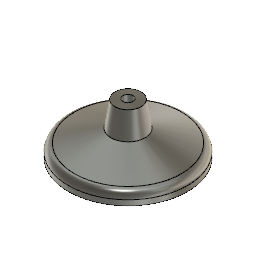
flag support (Autodesk Fusion 360 design; units mm, degrees)
Autodesk Fusion 360 part; units mm, degrees
sketch "Sketch1" plane through (0, 0, 0) normal (0, 1, 0) x (1, 0, 0)
  line L0 (0, -65) -> (0, 55)
  line L1 (-35, 24.9628) -> (-1, 24.9628)
  line L2 (-35, 24.9628) -> (-35, 21.7628)
  arc A0 (-35, 21.7628) -> (-31.4072, 17.5424) centre (-30.7249, 21.7628) ccw
  line L3 (-31.4072, 17.5424) -> (-10, 10)
  line L4 (-10, 10) -> (-7.7084, -4.6955)
  line L5 (0, -5) -> (-3, -5) construction
  line L6 (-7.7084, -4.6955) -> (-3, -5)
  line L7 (-3, -5) -> (-3, 20)
  line L8 (-1, 24.9628) -> (-1, 20)
  line L9 (-1, 20) -> (-3, 20)
  dimension "d1" = 34
  dimension "d2" = 3.2
  dimension "d3" = 3
  constraint vertical L0
  constraint perpendicular L0 L1
  constraint perpendicular L1 L2
  constraint tangent L2 A0
  constraint midpoint L0 L5.start
  constraint perpendicular L0 L5
  constraint perpendicular L5 L7
  constraint perpendicular L1 L8
  constraint perpendicular L7 L9
  measures "d1" distance of L1.start L1.end
  measures "d2" distance of L1.start L2.end
  measures "d3" distance of L5.start L5.end
revolve "Revolve1" add sketch "Sketch1" angle 360 about axis through (0, 0, 65) along (0, 0, -1)
